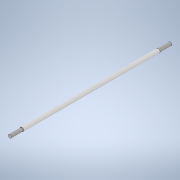
# Autodesk Inventor part: Barra de deslizamiento
Saved by Autodesk Inventor 2021 (Build 250183000, 183)
## iProperties
Created: 2021-05-29
Part Number: Barra de deslizamiento
Material: Generic
Document SubType Name: Modeling
Designer: Nelson
Density: 1 g/cm^3
Appearance: Default
Author: Nelson
Autodesk Inventor part; units mm, degrees
ref_plane "YZ Plane" through (0, 0, 0) normal (1, 0, 0) x (0, 1, 0)
ref_plane "XZ Plane" through (0, 0, 0) normal (0, 1, 0) x (-1, 0, 0)
ref_plane "XY Plane" through (0, 0, 0) normal (0, 0, 1) x (1, 0, 0)
sketch "Sketch3" plane through (0, 0, 0) normal (1, 0, 0) x (0, 1, 0)
  line L0 (0, 0) -> (11.1125, 0)
  line L1 (11.1125, 0) -> (11.1125, -80)
  line L2 (11.1125, -80) -> (12.7, -80)
  line L3 (12.7, -80) -> (12.7, -1000)
  line L4 (12.7, -1000) -> (11.1125, -1000)
  line L5 (11.1125, -1000) -> (11.1125, -1080)
  line L6 (11.1125, -1080) -> (0, -1080)
  line L7 (0, 0) -> (0, -1080)
  dimension "d7" = 11.1125
  dimension "d8" = 80
  dimension "d9" = 1.5875
  dimension "d10" = 920
  dimension "d11" = 1.5875
  dimension "d12" = 80
  dimension "d13" = 11.1125
  constraints: 16 end point, 4 perpendicular, 2 horizontal, 1 vertical
  measures "d7" distance of L0.start L0.end
  measures "d8" distance of L0.end L1.end
  measures "d9" distance of L1.end L2.end
  measures "d10" distance of L2.end L3.end
  measures "d11" distance of L3.end L4.end
  measures "d12" distance of L4.end L5.end
  measures "d13" distance of L5.end L6.end
revolve "Revolution1" add sketch "Sketch3" angle 360 about axis through (0, 0, 0) along (0, 0, -1)
thread "Thread3" size "7/8-9 UNC" class "2A" standard "ANSI Unified Screw Threads" full length
thread "Thread4" size "7/8-9 UNC" class "2A" standard "ANSI Unified Screw Threads" length 80
equation "\"d11\" = d9"
equation "\"d12\" = d8"
equation "\"d13\" = d7"
body "Solid2"
